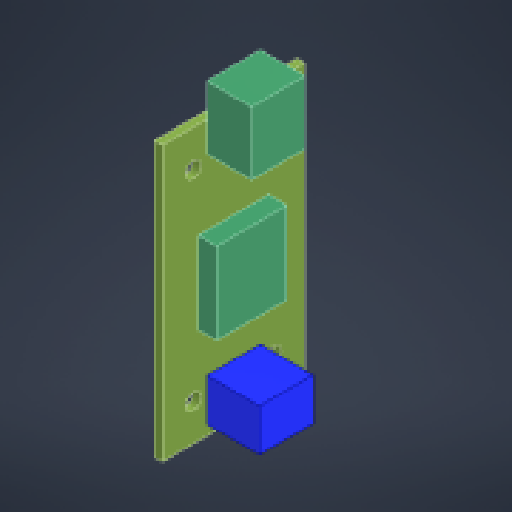
# Autodesk Inventor part: buck_converter
Saved by Autodesk Inventor 2025 (Build 290162000, 162)
## iProperties
Created: 2024-09-04
Part Number: buck_converter
Material: Generic
Document SubType Name: Modeling
Designer: Dawid
Density: 1 g/cm^3
Appearance: Default
Author: Dawid
Autodesk Inventor part; units mm, degrees
ref_plane "YZ Plane" through (0, 0, 0) normal (1, 0, 0) x (0, 1, 0)
ref_plane "XZ Plane" through (0, 0, 0) normal (0, 1, 0) x (-1, 0, 0)
ref_plane "XY Plane" through (0, 0, 0) normal (0, 0, 1) x (1, 0, 0)
sketch "Sketch1" plane through (0, 0, 0) normal (1, 0, 0) x (0, 1, 0)
  line L0 (0, 0) -> (52, 0)
  line L1 (52, 0) -> (52, -23)
  line L2 (52, -23) -> (0, -23)
  line L3 (0, -23) -> (0, 0)
  circle A0 centre (45.05, -3.88) radius 1.5
  circle A1 centre (45.05, -19.12) radius 1.5
  circle A2 centre (6.95, -3.88) radius 1.5
  circle A3 centre (6.95, -19.12) radius 1.5
  line L4 (45.05, -3.88) -> (6.95, -19.12) construction
  point P0 (26, -11.5)
  point P1 (52, -11.5)
  point P2 (26, 0)
  dimension "d0" = 23
  dimension "d1" = 52
  dimension "d2" = 3
  dimension "d3" = 15.24
  dimension "d4" = 38.1
  constraints: 10 end point, 4 centre point, 3 equal radius, 3 horizontal alignment, 3 midpoint, 3 vertical alignment, 2 parallel, 1 horizontal, 1 perpendicular
  measures "d0" distance of L0.end L1.end
  measures "d1" distance of L1.end L2.end
  measures "d2" diameter of A0
  measures "d3" distance of A1.centre L4.start
  measures "d4" distance of L4.end A1.centre
extrude "Extrusion1" add sketch "Sketch1" along normal blind 1.5
sketch "Sketch2" plane through (1.5, 0, 0) normal (1, 0, 0) x (0, 0, -1)
  line L0 (23, 0) -> (23, 52) construction
  line L1 (23, 52) -> (0, 52) construction
  line L2 (0, 52) -> (0, 0) construction
  line L3 (0, 0) -> (23, 0) construction
  circle A0 centre (19.12, 6.95) radius 1.5 construction
  circle A1 centre (3.88, 6.95) radius 1.5 construction
  circle A2 centre (19.12, 45.05) radius 1.5 construction
  circle A3 centre (3.88, 45.05) radius 1.5 construction
  line L4 (6.42, 58.32) -> (16.58, 58.32)
  line L5 (16.58, 58.32) -> (16.58, 46.32)
  line L6 (16.58, 46.32) -> (6.42, 46.32)
  line L7 (6.42, 46.32) -> (6.42, 58.32)
  line L8 (3.88, 45.05) -> (19.12, 45.05) construction
  point P0 (11.5, 45.05)
  point P1 (11.5, 46.32)
  dimension "d7" = 12
  dimension "d8" = 10.16
  dimension "d9" = 1.27
  constraints: 10 end point, 2 horizontal, 2 midpoint, 2 parallel, 1 perpendicular, 1 vertical alignment
  measures "d7" distance of L4.end L5.end
  measures "d8" distance of L5.end L6.end
  measures "d9" distance from line of L6 L8.start
extrude "Extrusion2" add sketch "Sketch2" along normal blind 8.5 separate body
sketch "Sketch3" plane through (1.5, 0, 0) normal (1, 0, 0) x (0, 0, -1)
  circle A0 centre (3.88, 6.95) radius 1.5 construction
  circle A1 centre (19.12, 6.95) radius 1.5 construction
  line L0 (0, 0) -> (23, 0) construction
  line L1 (6.42, 9.95) -> (16.58, 9.95)
  line L2 (16.58, 9.95) -> (16.58, 1.95)
  line L3 (16.58, 1.95) -> (6.42, 1.95)
  line L4 (6.42, 1.95) -> (6.42, 9.95)
  line L5 (3.88, 6.95) -> (19.12, 6.95) construction
  point P0 (11.5, 6.95)
  point P1 (11.5, 9.95)
  dimension "d12" = 10.16
  dimension "d13" = 8
  dimension "d14" = 3
  constraints: 10 end point, 2 horizontal, 2 midpoint, 2 parallel, 1 perpendicular, 1 vertical alignment
  measures "d12" distance of L2.end L3.end
  measures "d13" distance of L1.end L2.end
  measures "d14" distance from line of L1 L5.start
extrude "Extrusion3" add sketch "Sketch3" along normal blind 10 separate body
sketch "Sketch4" plane through (1.5, 0, 0) normal (1, 0, 0) x (0, 0, -1)
  circle A0 centre (3.88, 45.05) radius 1.5 construction
  circle A1 centre (19.12, 6.95) radius 1.5 construction
  line L0 (4.8192, 33.7605) -> (18.1808, 33.7605)
  line L1 (18.1808, 33.7605) -> (18.1808, 18.2395)
  line L2 (18.1808, 18.2395) -> (4.8192, 18.2395)
  line L3 (4.8192, 18.2395) -> (4.8192, 33.7605)
  line L4 (3.88, 45.05) -> (19.12, 6.95) construction
  point P0 (0, 0)
  point P1 (18.1808, 26)
  point P2 (11.5, 26)
  point P3 (11.5, 33.7605)
  constraints: 10 end point, 3 midpoint, 2 parallel, 1 horizontal, 1 horizontal alignment, 1 perpendicular, 1 vertical alignment
extrude "Extrusion4" add sketch "Sketch4" along normal blind 3.5 separate body
body "Solid1"
body "Solid2"
body "Solid3"
body "Solid4"
